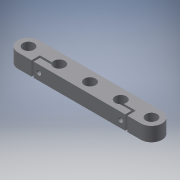
# Autodesk Inventor part: guide rod mount
Saved by Autodesk Inventor 2016 (Build 200138000, 138)
## iProperties
Created: 2017-08-15
Part Number: guide rod mount
Material: Generic
Document SubType Name: Modeling
Designer: zimirken
Density: 1 g/cm^3
Appearance: Default
Author: zimirken
Autodesk Inventor part; units mm, degrees
ref_plane "YZ Plane" through (0, 0, 0) normal (1, 0, 0) x (0, 1, 0)
ref_plane "XZ Plane" through (0, 0, 0) normal (0, 1, 0) x (-1, 0, 0)
ref_plane "XY Plane" through (0, 0, 0) normal (0, 0, 1) x (1, 0, 0)
sketch "Sketch1" plane through (0, 0, 0) normal (0, 0, 1) x (1, 0, 0)
  circle A0 centre (0, 0) radius 4
  circle A1 centre (43.5, 0) radius 4
  circle A2 centre (22, 0) radius 4
  line L0 (0, 0) -> (43.5, 0) construction
  line L1 (0, -7.5) -> (43.5, -7.5)
  line L2 (43.5, 7.5) -> (0, 7.5)
  arc A3 (0, 7.5) -> (0, -7.5) centre (0, 0) ccw
  arc A4 (43.5, -7.5) -> (43.5, 7.5) centre (43.5, 0) ccw
  point P0 (21.75, 0)
  dimension "d1" = 8
  dimension "d2" = 8
  dimension "d4" = 15
  dimension "d19" = 43.5
  dimension "d22" = 22
  constraints: 8 end point, 5 centre point, 4 point on circle, 4 tangent, 1 coincident, 1 equal radius, 1 horizontal, 1 midpoint, 1 parallel, 1 point on line
  measures "d1" diameter of A0
  measures "d2" diameter of A2
  measures "d4" distance between parallel lines of L1 L2
  measures "d19" distance of L0.start L0.end
  measures "d22" distance of A2.centre point (0, 0)
extrude "Extrusion1" add sketch "Sketch1" along normal blind 10
sketch "Sketch2" plane through (0, 0, 10) normal (0, 0, 1) x (1, 0, 0)
  line L0 (24.6458, -1.5) -> (34.1458, -1.5)
  line L1 (34.1458, -1.5) -> (34.1458, -3)
  line L2 (34.1458, -3) -> (24.6458, -3)
  line L3 (24.6458, -3) -> (24.6458, -1.5)
  line L4 (0, -7.5) -> (43.5, -7.5) projected
  line L5 (34.1458, -3) -> (32.6458, -3)
  line L6 (32.6458, -3) -> (32.6458, -7.5)
  line L7 (32.6458, -7.5) -> (34.1458, -7.5)
  line L8 (34.1458, -7.5) -> (34.1458, -3)
  circle A0 centre (22, 0) radius 4 construction
  point P0 (0, 0)
  dimension "d7" = 1.5
  dimension "d8" = 8
  dimension "d9" = 1.5
  dimension "d18" = 1
  constraints: 16 end point, 4 parallel, 2 horizontal, 2 perpendicular, 1 point on line, 2 other
  measures "d7" distance of L0.end L1.end
  measures "d8" distance from line of L2.end L6
  measures "d9" distance between parallel lines of L8 L6
extrude "Extrusion2" cut sketch "Sketch2" against normal through all
sketch "Sketch3" plane through (0, -7.5, 0) normal (0, -1, 0) x (1, 0, 0)
  line L0 (24.6458, 0) -> (32.6458, 0) construction
  line L1 (24.6458, 10) -> (24.6458, 0) construction
  line L2 (32.6458, 10) -> (24.6458, 10) construction
  line L3 (32.6458, 10) -> (32.6458, 0) construction
  line L4 (32.6458, 5) -> (25.7081, 5) construction
  line L5 (25.7081, 0) -> (25.7081, 10) construction
  circle A0 centre (29.1769, 5) radius 1.75
  point P0 (0, 0)
  dimension "d12" = 3.5
  constraints: 2 end point, 2 midpoint, 1 centre point, 2 other
  measures "d12" diameter of A0
extrude "Extrusion3" cut sketch "Sketch3" against normal through all
sketch "Sketch4" plane through (0, 7.5, 0) normal (0, 1, 0) x (1, 0, 0)
  circle A0 centre (29.1769, -5) radius 1.75 construction
  line L0 (30.7935, -2.2) -> (32.4101, -5)
  line L1 (32.4101, -5) -> (30.7935, -7.8)
  line L2 (30.7935, -7.8) -> (27.5603, -7.8)
  line L3 (27.5603, -7.8) -> (25.9438, -5)
  line L4 (25.9438, -5) -> (27.5603, -2.2)
  line L5 (27.5603, -2.2) -> (30.7935, -2.2)
  point P0 (0, 0)
  dimension "d15" = 5.6
  constraints: 12 end point, 1 coincident, 1 horizontal, 13 other
  measures "d15" distance between parallel lines of L2 L5
extrude "Extrusion4" cut sketch "Sketch4" against normal blind 3
mirror "Mirror1" about plane through (0, 0, 0) normal (1, 0, 0) of "Extrusion1", "Extrusion2", "Extrusion3", "Extrusion4"
body "Solid1"
